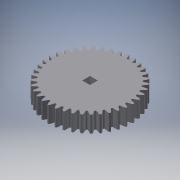
# Autodesk Inventor part: gear 3 shaft
Saved by Autodesk Inventor 2017 (Build 210142000, 142)
## iProperties
Created: 2018-04-17
Part Number: gear 3 shaft
Material: Generic
Document SubType Name: Modeling
Designer: RKL
Density: 1 g/cm^3
Appearance: Default
Author: RKL
Autodesk Inventor part; units mm, degrees
ref_plane "YZ Plane" through (0, 0, 0) normal (1, 0, 0) x (0, 1, 0)
ref_plane "XZ Plane" through (0, 0, 0) normal (0, 1, 0) x (-1, 0, 0)
ref_plane "XY Plane" through (0, 0, 0) normal (0, 0, 1) x (1, 0, 0)
sketch "Sketch1" plane through (0, 0, 0) normal (0, 0, 1) x (1, 0, 0)
  spline S0 degree 3 poles (-3.2895, 51.1443) (-3.0035, 50.6321) (-2.5744, 49.8638) (-2.0953, 48.7925) (-1.7794, 47.9717) (-1.4976, 47.137) (-1.371, 46.4122) (-1.1673, 45.9371) (-0.9981, 45.6962) (-0.8344, 45.5474) (-0.6488, 45.4276) (-0.369, 45.3295) (0, 45.3347) (0.369, 45.3295) (0.6488, 45.4276) (0.8344, 45.5474) (0.9981, 45.6962) (1.1673, 45.9371) (1.371, 46.4122) (1.4976, 47.137) (1.7794, 47.9717) (2.0953, 48.7925) (2.5744, 49.8638) (3.0035, 50.6321) (3.2895, 51.1443) knots 0 0 0 0 0.175874 0.263832 0.351787 0.439736 0.527671 0.571516 0.593484 0.61547 0.637423 0.659417 0.703249 0.747082 0.769075 0.791029 0.813015 0.834983 0.878827 0.966763 1.054712 1.142666 1.230624 1.406499 1.406499 1.406499 1.406499
  circle A0 centre (0, 0) radius 45.3326 construction
  circle A1 centre (0, 0) radius 45.81 construction
  circle A2 centre (0, 0) radius 48.75 construction
  circle A3 centre (0, 0) radius 51.25
  point P0 (-2.4624, 49.5922)
  point P1 (-2.1025, 48.7896)
  point P2 (-1.7851, 47.9693)
  point P3 (-1.5192, 47.131)
  point P4 (-1.3016, 46.279)
  point P5 (-1.1207, 45.8796)
  point P6 (-0.992, 45.7016)
  point P7 (-0.8307, 45.5522)
  point P8 (-0.6448, 45.4354)
  point P9 (-0.4373, 45.3625)
  point P10 (0, 45.3326)
  point P11 (0.4373, 45.3625)
  point P12 (0.6448, 45.4354)
  point P13 (0.8307, 45.5522)
  point P14 (0.992, 45.7016)
  point P15 (1.1207, 45.8796)
  point P16 (1.3016, 46.279)
  point P17 (1.5192, 47.131)
  point P18 (1.7851, 47.9693)
  point P19 (2.1025, 48.7896)
  point P20 (2.4624, 49.5922)
  constraints: 4 centre point, 2 point on circle, 51 other
extrude "Extrusion1" add sketch "Sketch1" against normal blind 20
extrude "Extrusion2" cut sketch "Sketch1" against normal through all contours A3 S0 picked at (-0.2191, 49.0308)
pattern_circular "Circular Pattern1" count 39 over 360 about axis through (0, 0, 0) along (0, 0, -1) of "Extrusion2"
sketch "Sketch2" plane through (0, 0, 0) normal (0, 0, 1) x (1, 0, 0)
  line L0 (4.7625, -4.7625) -> (-4.7625, -4.7625)
  line L1 (-4.7625, -4.7625) -> (-4.7625, 4.7625)
  line L2 (-4.7625, 4.7625) -> (4.7625, 4.7625)
  line L3 (4.7625, 4.7625) -> (4.7625, -4.7625)
  line L4 (4.7625, -4.7625) -> (-4.7625, 4.7625) construction
  line L5 (-4.7625, -4.7625) -> (4.7625, 4.7625) construction
  point P0 (0, 0)
  dimension "d7" = 9.525
  constraints: 12 end point, 2 midpoint, 2 parallel, 2 perpendicular, 1 horizontal
  measures "d7" distance of L0.end L1.end
extrude "Extrusion3" cut sketch "Sketch2" against normal through all
equation "\"d0\" = FaceWidth"
equation "\"Module\" = 2.5"
equation "\"PressureAngle\" = 20deg"
equation "\"UnitProfileClearance\" = 0.25"
equation "\"UnitRoundRadius\" = 0.35"
equation "\"HeadDiameter\" = 102.5"
equation "\"RootDiameter\" = 90.66524"
equation "\"BaseDiameter\" = 91.62003"
equation "\"PitchDiameter\" = 97.5"
equation "\"FaceWidth\" = 20"
equation "\"HelixAngle\" = 0"
equation "\"UnitCorrection\" = 0"
equation "\"UnitAddendumModification\" = 0"
equation "\"CircularPitch\" = 7.853982"
equation "\"UnitBacklashShift\" = -0.116952"
equation "\"TotalToolShift\" = -0.29238"
equation "\"IsInternal\" = 0"
body "Solid1"
